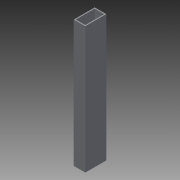
# Autodesk Inventor part: Waveguide Terminator
Saved by Autodesk Inventor 2014 (Build 180170000, 170)
## iProperties
Created: 2014-05-15
Part Number: Waveguide Terminator
Material: Generic
Document SubType Name: Modeling
Designer: ijs09
Density: 1 g/cm^3
Appearance: Default
Author: ijs09
Autodesk Inventor part; units mm, degrees
ref_plane "YZ Plane" through (0, 0, 0) normal (1, 0, 0) x (0, 1, 0)
ref_plane "XZ Plane" through (0, 0, 0) normal (0, 1, 0) x (-1, 0, 0)
ref_plane "XY Plane" through (0, 0, 0) normal (0, 0, 1) x (1, 0, 0)
sketch "Sketch1" plane through (0, 0, 0) normal (0, 0, 1) x (1, 0, 0)
  line L0 (5.7625, -10.525) -> (-5.7625, -10.525)
  line L1 (-5.7625, -10.525) -> (-5.7625, 10.525)
  line L2 (-5.7625, 10.525) -> (5.7625, 10.525)
  line L3 (5.7625, 10.525) -> (5.7625, -10.525)
  point P0 (0, 0)
  dimension "d2" = 21.05
  dimension "d4" = 10.525
  dimension "d7" = 11.525
  dimension "d8" = 5.7625
  constraints: 8 end point, 2 parallel, 1 horizontal, 1 perpendicular
  measures "d2" distance between parallel lines of L0 L2
  measures "d4" distance from line of point (0, 0) L2
  measures "d7" distance between parallel lines of L1 L3
  measures "d8" distance from line of L1 point (0, 0)
extrude "Extrusion1" add sketch "Sketch1" against normal blind 127
sketch "Sketch2" plane through (0, 0, 0) normal (0, 0, 1) x (1, 0, 0)
  line L0 (5.7625, -10.525) -> (-5.7625, -10.525) projected
  line L1 (5.7625, 10.525) -> (5.7625, -10.525) projected
  line L2 (-5.7625, 10.525) -> (5.7625, 10.525) projected
  line L3 (-5.7625, -10.525) -> (-5.7625, 10.525) projected
  line L4 (-4.7625, 9.525) -> (4.7625, 9.525)
  line L5 (4.7625, 9.525) -> (4.7625, -9.525)
  line L6 (4.7625, -9.525) -> (-4.7625, -9.525)
  line L7 (-4.7625, -9.525) -> (-4.7625, 9.525)
  point P0 (0, 0)
  dimension "d11" = 1
  dimension "d12" = 1
  dimension "d13" = 1
  dimension "d14" = 1
  constraints: 8 end point, 2 parallel, 1 horizontal, 1 perpendicular
  measures "d11" distance between parallel lines of L2 L4
  measures "d12" distance between parallel lines of L3 L7
  measures "d13" distance between parallel lines of L0 L6
  measures "d14" distance between parallel lines of L1 L5
extrude "Extrusion2" cut sketch "Sketch2" against normal blind 125 contours L4 L5 L6 L7
equation "\"d2\" = 2 * d4"
equation "\"d8\" = 0.5 * d7"
equation "\"d12\" = d11"
equation "\"d13\" = d11"
equation "\"d14\" = d11"
body "Solid1"
